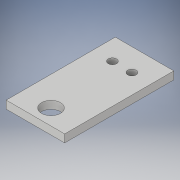
# Autodesk Inventor part: Side Attatchment
Saved by Autodesk Inventor 2019 (Build 230136000, 136)
## iProperties
Created: 2019-01-05
Part Number: Side Attatchment
Material: Generic
Document SubType Name: Modeling
Designer: ashle
Density: 1 g/cm^3
Appearance: Default
Author: ashle
Autodesk Inventor part; units mm, degrees
ref_plane "YZ Plane" through (0, 0, 0) normal (1, 0, 0) x (0, 1, 0)
ref_plane "XZ Plane" through (0, 0, 0) normal (0, 1, 0) x (-1, 0, 0)
ref_plane "XY Plane" through (0, 0, 0) normal (0, 0, 1) x (1, 0, 0)
sketch "Sketch2" plane through (0, 0, 0) normal (0, 1, 0) x (-1, 0, 0)
  line L0 (15, 28) -> (-15, 28)
  line L1 (-15, 28) -> (-15, -28)
  line L2 (-15, -28) -> (15, -28)
  line L3 (15, -28) -> (15, 28)
  line L4 (0, 0) -> (0, -28) construction
  line L5 (0, 0) -> (0, 28) construction
  line L6 (0, 0) -> (15, 0) construction
  line L7 (0, 0) -> (-15, 0) construction
  dimension "d45" = 30
  dimension "d46" = 56
  constraints: 16 end point, 4 midpoint, 2 collinear, 2 parallel, 1 horizontal, 1 perpendicular
  measures "d45" distance of L0.start L0.end
  measures "d46" distance of L2.end L0.start
extrude "Main Body Sketch" add sketch "Sketch2" along normal blind 4
ref_plane "Work Plane1" through (0, 4, 0) normal (0, 1, 0) x (1, 0, 0)
sketch "Sketch4" plane through (0, 4, 0) normal (0, 1, 0) x (1, 0, 0)
  circle A0 centre (0, -20) radius 4.8537
  line L0 (15, 28) -> (-15, 28) projected
  line L1 (-15, 28) -> (-15, -28) projected
  circle A1 centre (5, 16.5) radius 2.15
  circle A2 centre (-5, 16.5) radius 2.15
  line L2 (15, -28) -> (15, 28) projected
  dimension "d84" = 48
  dimension "d85" = 30
  dimension "d86" = 15
  dimension "d87" = 4.3
  dimension "d88" = 4.3
  dimension "d89" = 10
  dimension "d90" = 10
  dimension "d91" = 11.5
  dimension "d92" = 11.5
  constraints: 3 centre point
  measures "d84" distance from line of L0 A0.centre
  measures "d85" distance of L0.start L0.end
  measures "d86" distance from line of L1 A0.centre
  measures "d87" diameter of A1
  measures "d88" diameter of A2
  measures "d89" distance from line of L2 A1.centre
  measures "d90" distance of A2.centre A1.centre
  measures "d91" distance from line of L0 A1.centre
  measures "d92" distance from line of L0 A2.centre
extrude "Holes Cuts" cut sketch "Sketch4" against normal up to surface (4 mm away)
equation "\"d46\" = AH"
equation "\"AH\" = 56"
equation "\"BD\" = 4"
body "Solid1"
